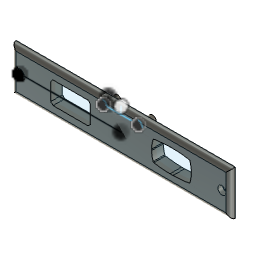
obere heckplatte v6 (Autodesk Fusion 360 design; units mm, degrees)
Autodesk Fusion 360 part; units mm, degrees
sketch "Skizze1" plane through (0, 0, 0) normal (0, 1, 0) x (1, 0, 0)
  line L0 (0, 0) -> (94, 0)
  line L1 (0, 0) -> (0, -19)
  line L2 (0, -19) -> (94, -19)
  line L3 (94, -19) -> (94, 0)
  dimension "d1" = 94
  dimension "d2" = 19
  constraint coincident L0.start L1.start
  constraint horizontal L0
  constraint perpendicular L0 L1
  constraint perpendicular L1 L2
  constraint perpendicular L0 L3
  measures "d1" distance of L0.start L0.end
  measures "d2" distance of L0.start L1.end
extrude "Extrusion1" add sketch "Skizze1" along normal blind 2
sketch "Skizze2" plane through (0, 0, 0) normal (0, -1, 0) x (1, 0, 0)
  line L0 (0, 19) -> (0, 0)
  line L1 (0, 0) -> (94, 0)
  line L2 (94, 0) -> (94, 19)
  line L3 (94, 19) -> (0, 19)
  circle A0 centre (3.75, 9.5) radius 1.75
  circle A1 centre (90.25, 9.5) radius 1.75
  dimension "d8" = 3.5
  dimension "d9" = 3.5
  measures "d8" diameter of A0
  measures "d9" diameter of A1
extrude "Extrusion2" cut sketch "Skizze2" against normal blind 2 contours A0 | A1
fillet "Abrundung1" radius 2 4 edges at (47, 0, 19) (94, 0, 9.5) (47, 0, 0) (0, 0, 9.5)
sketch "Skizze3" plane through (0, 0, 0) normal (0, -1, 0) x (1, 0, 0)
  circle A0 centre (90.25, 9.5) radius 1.75
  line L0 (92, 9.5) -> (92, 17)
  line L1 (92, 17) -> (2, 17)
  line L2 (2, 17) -> (2, 9.5)
  circle A1 centre (3.75, 9.5) radius 1.75
  line L3 (2, 9.5) -> (2, 2)
  line L4 (2, 2) -> (92, 2)
  line L5 (92, 2) -> (92, 9.5)
  line L6 (3.75, 9.5) -> (47, 9.5)
  line L7 (47, 19) -> (47, 18)
  line L8 (47, 18) -> (47, 16)
  line L9 (47, 16) -> (54.56, 16)
  line L10 (47, 16) -> (39.5, 16)
  circle A2 centre (39.5, 16) radius 1.55
  circle A3 centre (54.56, 16) radius 1.55
  dimension "d14" = 43.25
  dimension "d15" = 1
  dimension "d16" = 2
  dimension "d17" = 7.56
  dimension "d18" = 7.5
  dimension "d19" = 3.1
  dimension "d20" = 3.1
  constraint coincident A1.centre L6.start
  constraint perpendicular L2 L6
  constraint perpendicular L1 L7
  constraint perpendicular L1 L8
  constraint perpendicular L8 L9
  constraint perpendicular L8 L10
  constraint coincident L10.end A2.centre
  constraint coincident L9.end A3.centre
  measures "d14" distance of A1.centre L6.end
  measures "d15" distance of L7.start L7.end
  measures "d16" distance of L7.end L8.end
  measures "d17" distance of L8.end L9.end
  measures "d18" distance of L8.end L10.end
  measures "d19" diameter of A2
  measures "d20" diameter of A3
sketch "Skizze4" plane through (0, 2, 0) normal (0, 1, 0) x (-1, 0, 0)
  circle A0 centre (-90.25, 9.5) radius 1.75
  circle A1 centre (-3.75, 9.5) radius 1.75
  line L0 (0, 0) -> (0, 19)
  line L1 (0, 19) -> (-94, 19)
  line L2 (-94, 19) -> (-94, 0)
  line L3 (-94, 0) -> (0, 0)
  line L4 (-47, 19) -> (-47, 15)
  line L5 (-47, 15) -> (-39.5, 15)
  line L6 (-47, 15) -> (-54.5, 15)
  circle A2 centre (-39.5, 15) radius 1.55
  circle A3 centre (-54.5, 15) radius 1.55
  dimension "d21" = 4
  dimension "d22" = 7.5
  dimension "d23" = 7.5
  dimension "d24" = 3.1
  dimension "d25" = 3.1
  constraint midpoint L1 L4.start
  constraint perpendicular L1 L4
  constraint perpendicular L4 L5
  constraint perpendicular L4 L6
  constraint coincident L5.end A2.centre
  constraint coincident L6.end A3.centre
  measures "d21" distance of L4.start L4.end
  measures "d22" distance of L4.end L5.end
  measures "d23" distance of L4.end L6.end
  measures "d24" diameter of A2
  measures "d25" diameter of A3
extrude "Extrusion3" add sketch "Skizze4" along normal blind 4 contours A2 | A3
sketch "Skizze5" plane through (0, 2, 0) normal (0, 1, 0) x (-1, 0, 0)
  circle A0 centre (-54.5, 15) radius 1.55
  circle A1 centre (-39.5, 15) radius 1.55
  circle A2 centre (-90.25, 9.5) radius 1.75
  circle A3 centre (-3.75, 9.5) radius 1.75
  line L0 (0, 0) -> (0, 19)
  line L1 (0, 19) -> (-94, 19)
  line L2 (-94, 19) -> (-94, 0)
  line L3 (-94, 0) -> (0, 0)
  line L4 (-39.5, 15) -> (-39.5, 18)
  dimension "d28" = 3
  constraint coincident A1.centre L4.start
  constraint vertical L4
  measures "d28" distance of A1.centre L4.end
sketch "Skizze6" plane through (0, 0, 0) normal (0, -1, 0) x (1, 0, 0)
sketch "Skizze7" plane through (0, 0, 0) normal (0, -1, 0) x (1, 0, 0)
sketch "Skizze8" plane through (0, 0, 0) normal (0, -1, 0) x (1, 0, 0)
sketch "Skizze9" plane through (0, 0, 0) normal (0, -1, 0) x (1, 0, 0)
  circle A0 centre (90.25, 9.5) radius 1.75
  line L0 (92, 9.5) -> (92, 17)
  line L1 (92, 17) -> (2, 17)
  line L2 (2, 17) -> (2, 9.5)
  circle A1 centre (3.75, 9.5) radius 1.75
  line L3 (2, 9.5) -> (2, 2)
  line L4 (2, 2) -> (92, 2)
  line L5 (92, 2) -> (92, 9.5)
  line L6 (3.75, 9.5) -> (47, 9.5)
  line L7 (47, 9.5) -> (68.625, 9.5)
  line L8 (77.125, 14.5) -> (60.125, 14.5)
  line L9 (60.125, 14.5) -> (60.125, 4.5)
  line L10 (60.125, 4.5) -> (77.125, 4.5)
  line L11 (77.125, 4.5) -> (77.125, 14.5)
  line L12 (77.125, 14.5) -> (60.125, 4.5) construction
  line L13 (60.125, 14.5) -> (77.125, 4.5) construction
  line L14 (60.125, 4.5) -> (60.825, 4.5)
  line L15 (60.825, 4.5) -> (60.825, 5.2)
  line L16 (60.825, 5.2) -> (60.125, 5.2)
  line L17 (60.125, 5.2) -> (60.125, 4.5)
  line L18 (77.125, 4.5) -> (76.425, 4.5)
  line L19 (76.425, 4.5) -> (76.425, 5.2)
  line L20 (76.425, 5.2) -> (77.125, 5.2)
  line L21 (77.125, 5.2) -> (77.125, 4.5)
  line L22 (77.125, 14.5) -> (76.425, 14.5)
  line L23 (76.425, 14.5) -> (76.425, 13.8)
  line L24 (76.425, 13.8) -> (77.125, 13.8)
  line L25 (77.125, 13.8) -> (77.125, 14.5)
  line L26 (60.125, 14.5) -> (60.825, 14.5)
  line L27 (60.825, 14.5) -> (60.825, 13.8)
  line L28 (60.825, 13.8) -> (60.125, 13.8)
  line L29 (60.125, 13.8) -> (60.125, 14.5)
  line L30 (68.625, 14.5) -> (68.625, 15.2)
  line L31 (77.125, 9.5) -> (77.825, 9.5)
  line L32 (68.625, 4.5) -> (68.625, 3.8)
  line L33 (60.125, 9.5) -> (59.425, 9.5)
  line L34 (60.825, 5.2) -> (60.7857, 5.3206)
  line L35 (60.7857, 13.6794) -> (60.825, 13.8)
  line L36 (60.825, 13.8) -> (60.9401, 13.8207)
  line L37 (76.3099, 13.8207) -> (76.425, 13.8)
  line L38 (76.425, 13.8) -> (76.4643, 13.6794)
  line L39 (76.4643, 5.3206) -> (76.425, 5.2)
  line L40 (76.425, 5.2) -> (76.3099, 5.1793)
  line L41 (60.825, 5.2) -> (60.9401, 5.1793)
  arc A2 (60.7857, 13.6794) -> (60.7857, 5.3206) centre (73.6225, 9.5) ccw
  arc A3 (76.4643, 5.3206) -> (76.4643, 13.6794) centre (63.6275, 9.5) ccw
  arc A4 (76.3099, 13.8207) -> (60.9401, 13.8207) centre (68.625, -28.9951) ccw
  arc A5 (60.9401, 5.1793) -> (76.3099, 5.1793) centre (68.625, 47.9951) ccw
  point P0 (68.625, 9.5)
  dimension "d29" = 43.25
  dimension "d30" = 21.625
  dimension "d31" = 17
  dimension "d32" = 10
  dimension "d33" = 0.7
  dimension "d34" = 0.7
  dimension "d35" = 0.7
  dimension "d36" = 0.7
  dimension "d37" = 0.7
  dimension "d38" = 0.7
  dimension "d39" = 0.7
  dimension "d40" = 0.7
  dimension "d41" = 0.7
  dimension "d42" = 0.7
  dimension "d43" = 0.7
  dimension "d44" = 0.7
  dimension "d45" = 13.5
  dimension "d46" = 13.5
  dimension "d47" = 43.5
  dimension "d48" = 43.5
  constraint coincident A1.centre L6.start
  constraint perpendicular L2 L6
  constraint parallel L6 L7
  constraint horizontal L8
  constraint perpendicular L8 L9
  constraint parallel L8 L10
  constraint parallel L9 L11
  constraint coincident L12 P0
  constraint coincident L13 P0
  constraint coincident P0 L7.end
  constraint horizontal L14
  constraint vertical L15
  constraint horizontal L16
  constraint vertical L17
  constraint horizontal L18
  constraint vertical L19
  constraint horizontal L20
  constraint vertical L21
  constraint horizontal L22
  constraint vertical L23
  constraint horizontal L24
  constraint vertical L25
  constraint horizontal L26
  constraint vertical L27
  constraint horizontal L28
  constraint vertical L29
  constraint midpoint L8 L30.start
  constraint perpendicular L8 L30
  constraint midpoint L11 L31.start
  constraint perpendicular L11 L31
  constraint midpoint L10 L32.start
  constraint perpendicular L10 L32
  constraint midpoint L9 L33.start
  constraint perpendicular L9 L33
  constraint coincident L33.end L35
  constraint coincident L33.end L34
  constraint tangent L35 A2
  constraint tangent L34 A2
  constraint coincident L31.end L38
  constraint coincident L31.end L39
  constraint tangent L38 A3
  constraint tangent L39 A3
  constraint coincident L30.end L36
  constraint coincident L30.end L37
  constraint tangent L36 A4
  constraint tangent L37 A4
  constraint coincident L32.end L41
  constraint coincident L32.end L40
  constraint tangent L41 A5
  constraint tangent L40 A5
  measures "d29" distance of A1.centre L6.end
  measures "d30" distance of L6.end P0
  measures "d31" distance of L9.end L10.end
  measures "d32" distance of L8.end L9.end
  measures "d33" distance of L9.end L14.end
  measures "d34" distance of L9.end L16.end
  measures "d35" distance of L10.end L18.end
  measures "d36" distance of L10.end L20.end
  measures "d37" distance of L8.start L22.end
  measures "d38" distance of L8.start L24.end
  measures "d39" distance of L8.end L26.end
  measures "d40" distance of L8.end L28.end
  measures "d41" distance of L30.start L30.end
  measures "d42" distance of L31.start L31.end
  measures "d43" distance of L32.start L32.end
  measures "d44" distance of L33.start L33.end
  measures "d45" radius of A2
  measures "d46" radius of A3
  measures "d47" radius of A4
  measures "d48" radius of A5
sketch "Skizze10" plane through (0, 0, 0) normal (0, -1, 0) x (1, 0, 0)
extrude "Extrusion4" cut sketch "Skizze9" against normal blind 4 contours L8 L9 L10 L11 L34 L35 L36 L37 L38 L39 L40 L41 A2 A3 A4 A5
fillet "Abrundung2" radius 0.4 4 edges at (60.825, 1, 5.2) (76.425, 1, 5.2) (76.425, 1, 13.8) (60.825, 1, 13.8)
sketch "Skizze11" plane through (0, 2, 0) normal (0, 1, 0) x (-1, 0, 0)
  circle A0 centre (-39.5, 15) radius 1.75
  circle A1 centre (-54.5, 15) radius 1.75
  dimension "d53" = 3.5
  dimension "d54" = 3.5
  measures "d53" diameter of A0
  measures "d54" diameter of A1
extrude "Extrusion5" add sketch "Skizze11" along normal blind 2
sketch "Skizze12" plane through (0, 0, 0) normal (0, -1, 0) x (1, 0, 0)
sketch "Skizze13" plane through (0, 0, 0) normal (0, -1, 0) x (1, 0, 0)
sketch "Skizze14" plane through (0, 0, 0) normal (0, -1, 0) x (1, 0, 0)
  arc A0 (61.0622, 5.1576) -> (67.9745, 4.5) centre (68.625, 47.9951) ccw
  arc A1 (60.7503, 5.431) -> (61.0622, 5.1576) centre (61.1317, 5.5515) ccw
  arc A2 (60.125, 9.2404) -> (60.7503, 5.431) centre (73.6225, 9.5) ccw
  line L0 (60.125, 9.2404) -> (60.125, 9.7596)
  arc A3 (60.7503, 13.569) -> (60.125, 9.7596) centre (73.6225, 9.5) ccw
  arc A4 (61.0622, 13.8424) -> (60.7503, 13.569) centre (61.1317, 13.4485) ccw
  arc A5 (67.9745, 14.5) -> (61.0622, 13.8424) centre (68.625, -28.9951) ccw
  line L1 (67.9745, 14.5) -> (69.2755, 14.5)
  arc A6 (76.1878, 13.8424) -> (69.2755, 14.5) centre (68.625, -28.9951) ccw
  arc A7 (76.4997, 13.569) -> (76.1878, 13.8424) centre (76.1183, 13.4485) ccw
  arc A8 (77.125, 9.7596) -> (76.4997, 13.569) centre (63.6275, 9.5) ccw
  line L2 (77.125, 9.7596) -> (77.125, 9.2404)
  arc A9 (76.4997, 5.431) -> (77.125, 9.2404) centre (63.6275, 9.5) ccw
  arc A10 (76.1878, 5.1576) -> (76.4997, 5.431) centre (76.1183, 5.5515) ccw
  arc A11 (69.2755, 4.5) -> (76.1878, 5.1576) centre (68.625, 47.9951) ccw
  line L3 (69.2755, 4.5) -> (67.9745, 4.5)
  circle A12 centre (90.25, 9.5) radius 1.75
  line L4 (92, 9.5) -> (92, 17)
  line L5 (92, 17) -> (2, 17)
  line L6 (2, 17) -> (2, 9.5)
  circle A13 centre (3.75, 9.5) radius 1.75
  line L7 (2, 9.5) -> (2, 2)
  line L8 (2, 2) -> (92, 2)
  line L9 (92, 2) -> (92, 9.5)
  line L10 (3.75, 9.5) -> (25.375, 9.5)
  line L11 (25.375, 9.5) -> (47, 9.5)
  line L12 (33.875, 14.25) -> (16.875, 14.25)
  line L13 (16.875, 14.25) -> (16.875, 4.75)
  line L14 (16.875, 4.75) -> (33.875, 4.75)
  line L15 (33.875, 4.75) -> (33.875, 14.25)
  line L16 (33.875, 14.25) -> (16.875, 4.75) construction
  line L17 (16.875, 14.25) -> (33.875, 4.75) construction
  line L18 (33.875, 14.25) -> (32.875, 14.25)
  line L19 (32.875, 14.25) -> (32.875, 13.25)
  line L20 (32.875, 13.25) -> (33.875, 13.25)
  line L21 (33.875, 13.25) -> (33.875, 14.25)
  line L22 (33.875, 4.75) -> (32.875, 4.75)
  line L23 (32.875, 4.75) -> (32.875, 5.75)
  line L24 (32.875, 5.75) -> (33.875, 5.75)
  line L25 (33.875, 5.75) -> (33.875, 4.75)
  line L26 (16.875, 4.75) -> (17.875, 4.75)
  line L27 (17.875, 4.75) -> (17.875, 5.75)
  line L28 (17.875, 5.75) -> (16.875, 5.75)
  line L29 (16.875, 5.75) -> (16.875, 4.75)
  line L30 (16.875, 14.25) -> (17.875, 14.25)
  line L31 (17.875, 14.25) -> (17.875, 13.25)
  line L32 (17.875, 13.25) -> (16.875, 13.25)
  line L33 (16.875, 13.25) -> (16.875, 14.25)
  line L34 (16.875, 13.25) -> (17.875, 14.25)
  line L35 (32.875, 14.25) -> (33.875, 13.25)
  line L36 (33.875, 5.75) -> (32.875, 4.75)
  line L37 (17.875, 4.75) -> (16.875, 5.75)
  point P0 (25.375, 9.5)
  dimension "d57" = 21.625
  dimension "d58" = 17
  dimension "d59" = 9.5
  dimension "d60" = 1
  dimension "d61" = 1
  dimension "d62" = 1
  dimension "d63" = 1
  dimension "d64" = 1
  dimension "d65" = 1
  dimension "d66" = 1
  dimension "d67" = 1
  constraint coincident A13.centre L10.start
  constraint perpendicular L6 L10
  constraint parallel L10 L11
  constraint horizontal L12
  constraint perpendicular L12 L13
  constraint parallel L12 L14
  constraint parallel L13 L15
  constraint coincident L16 P0
  constraint coincident L17 P0
  constraint coincident P0 L10.end
  constraint horizontal L18
  constraint vertical L19
  constraint horizontal L20
  constraint vertical L21
  constraint horizontal L22
  constraint vertical L23
  constraint horizontal L24
  constraint vertical L25
  constraint horizontal L26
  constraint vertical L27
  constraint horizontal L28
  constraint vertical L29
  constraint horizontal L30
  constraint vertical L31
  constraint horizontal L32
  constraint vertical L33
  measures "d57" distance of A13.centre P0
  measures "d58" distance of L13.end L14.end
  measures "d59" distance of L12.end L13.end
  measures "d60" distance of L12.start L18.end
  measures "d61" distance of L12.start L20.end
  measures "d62" distance of L14.end L22.end
  measures "d63" distance of L14.end L24.end
  measures "d64" distance of L13.end L26.end
  measures "d65" distance of L13.end L28.end
  measures "d66" distance of L12.end L30.end
  measures "d67" distance of L12.end L32.end
extrude "Extrusion6" cut sketch "Skizze14" against normal blind 2 contours L10 L11 L12 L13 L15 L19 L20 L31 L32 | L10 L11 L13 L14 L15 L23 L24 L27 L28 | L31 L32 L34 | L27 L28 L37 | L23 L24 L36 | L19 L20 L35
sketch "Skizze15" plane through (0, 2, 0) normal (0, 1, 0) x (-1, 0, 0)
  line L0 (-47, 10) -> (-47, 9.5)
  line L1 (-35, 9.5) -> (-35, 15)
  line L2 (-35, 15) -> (-16, 15)
  line L3 (-16, 15) -> (-16, 9.5)
  line L4 (-16, 9.5) -> (-16, 4)
  line L5 (-16, 4) -> (-35, 4)
  line L6 (-35, 4) -> (-35, 9.5)
  line L7 (-59, 9.5) -> (-59, 15)
  line L8 (-59, 15) -> (-78, 15)
  line L9 (-78, 15) -> (-78, 4)
  line L10 (-78, 4) -> (-59, 4)
  line L11 (-59, 4) -> (-59, 9.5)
  line L12 (-35, 9.5) -> (-36, 9.5)
  line L13 (-36, 9.5) -> (-36, 16)
  line L14 (-36, 16) -> (-15, 16)
  line L15 (-15, 16) -> (-15, 3)
  line L16 (-36, 9.5) -> (-36, 3)
  line L17 (-36, 3) -> (-15, 3)
  line L18 (-58, 16) -> (-58, 3)
  line L19 (-58, 3) -> (-79, 3)
  line L20 (-79, 3) -> (-79, 16)
  line L21 (-79, 16) -> (-58, 16)
  line L22 (-47, 9.5) -> (-47, 9)
  line L23 (-47, 10) -> (-35, 10)
  line L24 (-47, 9) -> (-35, 9)
  line L25 (-47, 10) -> (-59, 10)
  line L26 (-59, 9) -> (-47, 9)
  dimension "d70" = 0.5
  dimension "d74" = 5.5
  dimension "d75" = 1
  dimension "d76" = 0.5
  constraint vertical L0
  constraint perpendicular L1 L2
  constraint perpendicular L2 L3
  constraint parallel L3 L4
  constraint perpendicular L3 L5
  constraint perpendicular L7 L8
  constraint perpendicular L9 L10
  constraint perpendicular L1 L12
  constraint perpendicular L13 L14
  constraint perpendicular L15 L17
  constraint perpendicular L7 L19
  constraint perpendicular L19 L20
  constraint perpendicular L18 L21
  constraint parallel L0 L22
  constraint coincident L1 L23.end
  constraint perpendicular L1 L23
  constraint coincident L6 L24.end
  constraint perpendicular L6 L24
  constraint coincident L7 L25.end
  constraint perpendicular L7 L25
  constraint coincident L11 L26.start
  measures "d70" distance of L0.start L0.end
  measures "d74" distance of L2.end L3.end
  measures "d75" distance of L1.start L12.end
  measures "d76" distance of L0.end L22.end
extrude "Extrusion7" add sketch "Skizze15" along normal blind 3 contours L0 L13 L16 L22 L23 L24 | L0 L18 L22 L25 L26 | L1 L12 L13 L23 | L7 L11 L18 L25 L26 | L6 L12 L16 L24 | L1 L2 L3 L4 L5 L6 | L7 L8 L9 L10 L11
delete_face "Fläche löschen1" 2 faces at (73.4351, 2, 9.4135) (22.875, 2, 7.9167)
sketch "Skizze16" plane through (0, 5, 0) normal (0, 1, 0) x (-1, 0, 0)
  line L0 (-59, 15) -> (-78, 15)
  line L1 (-78, 15) -> (-78, 4)
  line L2 (-78, 4) -> (-59, 4)
  line L3 (-59, 4) -> (-59, 9)
  line L4 (-59, 9) -> (-47, 9)
  line L5 (-47, 9) -> (-35, 9)
  line L6 (-35, 9) -> (-35, 4)
  line L7 (-35, 4) -> (-16, 4)
  line L8 (-16, 4) -> (-16, 15)
  line L9 (-16, 15) -> (-35, 15)
  line L10 (-35, 15) -> (-35, 10)
  line L11 (-35, 10) -> (-59, 10)
  line L12 (-59, 10) -> (-59, 15)
  line L13 (-16.875, 13.25) -> (-16.875, 5.75)
  line L14 (-16.875, 5.75) -> (-17.875, 4.75)
  line L15 (-17.875, 4.75) -> (-32.875, 4.75)
  line L16 (-32.875, 4.75) -> (-33.875, 5.75)
  line L17 (-33.875, 5.75) -> (-33.875, 13.25)
  line L18 (-33.875, 13.25) -> (-32.875, 14.25)
  line L19 (-32.875, 14.25) -> (-17.875, 14.25)
  line L20 (-17.875, 14.25) -> (-16.875, 13.25)
  line L21 (-77.125, 9.2404) -> (-77.125, 9.7596)
  arc A0 (-76.4997, 13.569) -> (-77.125, 9.7596) centre (-63.6275, 9.5) ccw
  arc A1 (-76.1878, 13.8424) -> (-76.4997, 13.569) centre (-76.1183, 13.4485) ccw
  arc A2 (-69.2755, 14.5) -> (-76.1878, 13.8424) centre (-68.625, -28.9951) ccw
  line L22 (-69.2755, 14.5) -> (-67.9745, 14.5)
  arc A3 (-61.0622, 13.8424) -> (-67.9745, 14.5) centre (-68.625, -28.9951) ccw
  arc A4 (-60.7503, 13.569) -> (-61.0622, 13.8424) centre (-61.1317, 13.4485) ccw
  arc A5 (-60.125, 9.7596) -> (-60.7503, 13.569) centre (-73.6225, 9.5) ccw
  line L23 (-60.125, 9.7596) -> (-60.125, 9.2404)
  arc A6 (-60.7503, 5.431) -> (-60.125, 9.2404) centre (-73.6225, 9.5) ccw
  arc A7 (-61.0622, 5.1576) -> (-60.7503, 5.431) centre (-61.1317, 5.5515) ccw
  arc A8 (-67.9745, 4.5) -> (-61.0622, 5.1576) centre (-68.625, 47.9951) ccw
  line L24 (-67.9745, 4.5) -> (-69.2755, 4.5)
  arc A9 (-76.1878, 5.1576) -> (-69.2755, 4.5) centre (-68.625, 47.9951) ccw
  arc A10 (-76.4997, 5.431) -> (-76.1878, 5.1576) centre (-76.1183, 5.5515) ccw
  arc A11 (-77.125, 9.2404) -> (-76.4997, 5.431) centre (-63.6275, 9.5) ccw
  line L25 (-35, 10) -> (-35, 9)
  line L26 (-59, 10) -> (-59, 9)
  constraint coincident L10.end L11.start
  constraint coincident L5.end L6.start
  constraint coincident L11.end L12.start
  constraint coincident L3.end L4.start
extrude "Extrusion8" cut sketch "Skizze16" against normal blind 1 contours L4 L5 L11 L25 L26
sketch "Skizze17" plane through (0, 0, 0) normal (0, -1, 0) x (1, 0, 0)
sketch "Skizze18" plane through (0, 2, 0) normal (0, 1, 0) x (-1, 0, 0)
  circle A0 centre (-54.5, 15) radius 1.6
  circle A1 centre (-39.5, 15) radius 1.6
  dimension "d81" = 3.2
  dimension "d82" = 3.2
  measures "d81" diameter of A0
  measures "d82" diameter of A1
extrude "Extrusion9" add sketch "Skizze18" along normal blind 4
